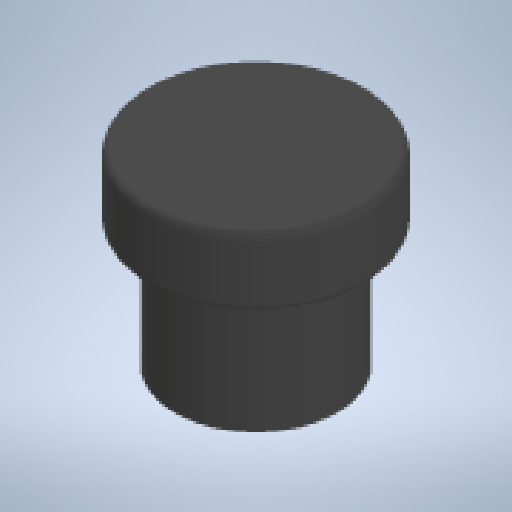
# Autodesk Inventor part: part7
Saved by Autodesk Inventor 2025.2 (Build 292293000, 293)
## iProperties
Created: 2024-12-09
Part Number: part7
Material: Kauczuk
Document SubType Name: Modeling
Designer: Marek
Density: 0.93 g/cm^3
Appearance: Kauczuk — czarny
Author: Marek
Autodesk Inventor part; units mm, degrees
ref_plane "YZ Plane" through (0, 0, 0) normal (1, 0, 0) x (0, 1, 0)
ref_plane "XZ Plane" through (0, 0, 0) normal (0, 1, 0) x (-1, 0, 0)
ref_plane "XY Plane" through (0, 0, 0) normal (0, 0, 1) x (1, 0, 0)
sketch "Szkic2" plane through (0, 0, 0) normal (1, 0, 0) x (0, 1, 0)
  line L0 (0, 0) -> (0, -6)
  line L1 (0, -6) -> (9, -6)
  line L2 (9, -6) -> (9, -8)
  line L3 (9, -8) -> (14, -8)
  line L4 (14, -8) -> (14, 0)
  line L5 (14, 0) -> (0, 0)
  dimension "d6" = 6
  dimension "d7" = 9
  dimension "d8" = 2
  dimension "d9" = 5
  constraints: 12 end point, 4 perpendicular, 2 vertical
  measures "d6" distance of L0.start L0.end
  measures "d7" distance of L0.end L1.end
  measures "d8" distance of L1.end L2.end
  measures "d9" distance of L2.end L3.end
revolve "Obrót1" add sketch "Szkic2" angle 360 about axis through (0, 14, 0) along (0, -1, 0)
sketch "Szkic3" plane through (0, 0, 0) normal (0, -1, 0) x (1, 0, 0)
  circle A0 centre (0, 0) radius 6 projected
  circle A1 centre (0, 0) radius 5.7
  dimension "d11" = 11.4
  constraints: 1 centre point, 1 coincident
  measures "d11" diameter of A1
extrude "Wyciągnięcie proste1" cut sketch "Szkic3" against normal blind 10 contours A1
fillet "Zaokrąglenie1" radius 0.5 2 edges at (0, 9, 8) (0, 14, 8)
